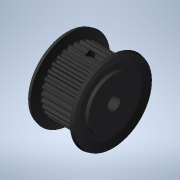
# Autodesk Inventor part: HTPA32S2M100-A-P4_a
Saved by Autodesk Inventor 2021 (Build 250183000, 183)
## iProperties
Created: 2025-04-04
Part Number: HTPA32S2M100-A-P4_a
Material: Generic
Catalog Web Link: www.cadenas.de
Description: HTPA_ _S2M040, HTPA_ _S2M060, HTPA_ _S2M100, HTPB_ _S2M040, HTPB_ _S2M060, HTPB_ _S2M100, HTPK_ _S2M040, HTPK_ _S2M060, HTPK_ _S2M100, HTPN_ _S2M040, HTPN_ _S2M060, HTPN_ _S2M100, HTPT_ _S2M040, HTPT_ _S2M060, HTPM_ _S2M040, HTPM_ _S2M060, HTPP_ _S2M040, HTPP_ _S2M060, HTPS_ _S2M040, HTPS_ _S2M060, HTPS_ _S2M100_a-High Torque Timing Pulleys S2M Type
Vendor: MISUMI
Document SubType Name: Modeling
Designer: psAdmin
Manufacturer: MISUMI
Mass: 4.25657 g
Surface Area: 28.5328 cm^2
Volume: 4.25657 cm^3
Density: 1 g/cm^3
Appearance: PSOLRGB-175-175-175
Category: PARTsolutions
Company: MISUMI
Title: HTPA32S2M100-A-P4
Author: Cadenas PARTsolutions
Comments: High Torque Timing Pulleys S2M Type
PSOL_IDENT_0: {$CADENAS_DATA/23d-libs/misumi/metric/51_timing_pulleys/htpm_s2m/htpa_s2m.prj},735 {VTYP=3D},{NB=HTP
PSOL_IDENT_1: A32S2M100-A-P4_a},{LINA=HTPA32S2M100-A-P4},{NN=HTPA_ _S2M040, HTPA_ _S2M060, HTPA_ _S2M100, HTPB_ _S
PSOL_IDENT_2: 2M040, HTPB_ _S2M060, HTPB_ _S2M100, HTPK_ _S2M040, HTPK_ _S2M060, HTPK_ _S2M100, HTPN_ _S2M040, HTP
PSOL_IDENT_3: N_ _S2M060, HTPN_ _S2M100, HTPT_ _S2M040, HTPT_ _S2M060, HTPM_ _S2M040, HTPM_ _S2M060, HTPP_ _S2M040
PSOL_IDENT_4: , HTPP_ _S2M060, HTPS_ _S2M040, HTPS_ _S2M060, HTPS_ _S2M100_a},{DATE=29.05.2023 09:16:33},{GEOMDATE=
PSOL_IDENT_5: 11.01.2023 01:57:31},{VERSION=},{LINEID=170},{WBVAR=MATP,ST,TNW,PS,SBS,DD,Z,J,Q,R,S,T,ALT1,ALT2,M,QS
PSOL_IDENT_6: C,QFC,QTC,ALT3,K,KSC,KFC,KTC,ALT4,ZM,ZSC,ZFC,ZTC,ALT5,ALT6,ALT7,FC,ALT8,SRG,ALT9,BTC,TL,ALT10,TPC,AL
PSOL_IDENT_7: T11,BC,ALT12,SLH,ALT13,BN},{WBNUMERIC=DD,Z,J,Q,R,S,T,QSC,QFC,QTC,K,KSC,KFC,KTC,ZSC,ZFC,ZTC,FC,SRG,BT
PSOL_IDENT_8: C,TL,BC,SLH,BN}  {NB=HTPA32S2M100-A-P4_a},{LINA=HTPA32S2M100-A-P4},{KT=DUMMY},{PN=HTPA32S2M100-A-P4}
PSOL_IDENT_9: ,{TYPE=HTPA},{MATP=A2017},{MATPALG= 'A2017','Aluminum Alloy 2000 series','S45CE','1045 Carbon Steel
PSOL_IDENT_10: Equivalent','SUS304','304 Stainless Steel' },{ST=CA},{STALG= 'CA' , 'Clear Anodize', 'BA','Black Ano
PSOL_IDENT_11: dize','HAT','Hard Clear Anodize' , 'ENP' , 'Electroless Nickel Plating' },{NT=32},{TNW=S2M100},{TNWA
PSOL_IDENT_12: LG= 'S2M040', 'S2M060','S2M100' },{BW=10},{PS=A},{PSALG='A','B'},{SBS=P},{SBSALG= 'H','Round Hole','
PSOL_IDENT_13: P','Round Hole + Tap','N','New JIS Keywayed Bore + Tap (Standard)','V','Stepped Hole','Y','Both Ends
PSOL_IDENT_14: Stepped Hole','WB','Double Stepped Hole' },{SHSA= 'H','Round Hole','P','Round Hole + Tap','N','New
PSOL_IDENT_15: JIS Keywayed Bore + Tap (Standard)','V','Stepped Hole','Y','Both Ends Stepped Hole','WB','Double Ste
PSOL_IDENT_16: pped Hole' },{SHSB='H','Round Hole','P','Round Hole + Tap','V','Stepped Hole','F','Stepped Hole (Cou
PSOL_IDENT_17: nterbore holes on the boss side)' },{SHSK='H','Round Hole','P','Round Hole + Tap'},{SBSPN=-P4},{DD=4
PSOL_IDENT_18: .00},{DDALG=[4:4/1],4.5,[5:6/1],6.35,[7:10/1]},{DDHA=[4:4/1],4.5,[5:6/1],6.35,[7:12/1]},{DDHBK=0},{D
PSOL_IDENT_19: DPA=[4:4/1],4.5,[5:6/1],6.35,[7:10/1]},{DDPBK=0},{DDNA=[8:8/1]},{DDNBK=0},{DDNK=0},{DDCA=0},{DDCBK=0
PSOL_IDENT_20: },{DDVA=[4:4/1],4.5,[5:6/1],6.35,[7:10/1]},{DDVF=0},{DDY=[4:10/1]},{DDWB=[4:8/1]},{Z=0},{ZALG=[0]},{
PSOL_IDENT_21: ZQRMIN=6},{ZAMAX=12},{ZBMAX=0},{DDZ=4},{J=0.0},{JALG=[0]},{JMAX=13},{JMIN=2},{JPN=},{QRMAX=12},{QRMI
PSOL_IDENT_22: N=6},{WBRMAX=-2.00},{WBQMIN=8},{Q=0},{QALG=[0]},{QPN=},{R=0},{RALG=[0]},{S=0.0},{SALG=[0]},{SPN=},{S
PSOL_IDENT_23: MAX=9},{T=0.0},{TALG=[0]},{TPN=},{TMAX=12},{A=11},{W=15},{L=0},{PD=20.37},{OD=19.86},{D=0},{DALG=12}
PSOL_IDENT_24: ,{DE=16},{F=25},{E=16},{BBK=0.000},{TTK=0.0},{TT=1},{WL=15.000},{ALT1=},{ALT1ALG= '','w/o KC90 (Set
PSOL_IDENT_25: Screw Angle)','KC90','with KC90 (Set Screw Angle)' },{ANG=123.750},{ALT1PN=},{ALT2=},{ALT2ALG= '','N
PSOL_IDENT_26: ot applicable' },{M=N/A},{MALG= 'N/A' },{MFTALG= 'N/A' },{MSALG= 'N/A' },{M3D=0.000},{KDML=0},{ML=0}
PSOL_IDENT_27: ,{MUL=0},{PITCH=0},{QSC=0.0},{QSCALG=0},{QFC=0.0},{QFCALG=0},{QTC=0.0},{QTCALG=0},{QPCDMIN=0},{QPCDM
PSOL_IDENT_28: INALG=0},{QPCDMAX=12},{ALT2PN=},{ALT3=},{ALT3ALG= '','Not applicable' },{K=0.0},{KALG=0},{KMIN=4},{K
PSOL_IDENT_29: FTMAX=0.0},{KSMAX=0.0},{KSC=0.0},{KSCALG=0},{KFC=0.0},{KFCALG=0},{KTC=0.0},{KTCALG=0},{KPCDMIN=8},{K
PSOL_IDENT_30: PCDMINALG=8},{KPCDMAX=12},{KSCMIN=8.0},{KSCMINALG=8},{ALT3PN=},{ALT4=},{ALT4ALG= '','Not applicable'
PSOL_IDENT_31: },{ALT4MIN=14.5},{ALT4MAX=5.5},{ZM=N/A},{ZMALG= 'N/A' },{ZMSALG= 'N/A' },{ZMFTALG= 'N/A' },{ZMDD1=0
PSOL_IDENT_32: .0},{ZMDD2=0.0},{ZMHH=0.0},{ZSC=0.0},{ZSCALG=[0]},{ZFC=0.0},{ZFCALG=[0]},{ZTC=0.0},{ZTCALG=[0]},{ZPC
PSOL_IDENT_33: DMIN=0},{ZPCDMINALG=0},{ZPCDMAX=12},{ALT4PN=},{ALT5=},{ALT5ALG= '','Flange Attached','NFC','with NFC
PSOL_IDENT_34: (Flange not Attached)' },{ALT5PN=},{ALT6=},{ALT6ALG= '','w/o Flange Attached on One Side Only','RFC'
PSOL_IDENT_35: ,'with RFC (Flange Attached on The Boss Side Only)','LFC','with LFC (Flange Attached on The Opposite
PSOL_IDENT_36: Side Only)' },{ALT6PN=},{ALT7=},{ALT7ALG= '','w/o FC (Flange Cut)','FC','with FC (Flange Cut)' },{F
PSOL_IDENT_37: C=0.0},{FCALG=0},{FCMIN=21.0},{FCMAX=23.0},{ALT7PN=},{ALT8=},{ALT8ALG= '','Not applicable' },{ALT8AL
PSOL_IDENT_38: GALG=12},{ALT8DD2=0},{ALT8MM=0},{ALT8NN=0},{QC=0},{KC=0},{ZC=0},{SRG=0.0},{SRGALG=[0]},{SRGMAX=0},{D
PSOL_IDENT_39: D2=0.0},{MM=0.00},{NN=0.00},{ALT8PN=},{ALT9ALG= '','w/o BTC (Taper for Bearing Holder)','BTC','with
PSOL_IDENT_40: BTC (Taper for Bearing Holder)' },{ALT9=},{BTC9=6},{TL9=1},{BTC=0},{BTCALG=[0]},{TL=0.0},{TLALG=[0]}
PSOL_IDENT_41: ,{TLMIN=1.0},{TLMAX=-15.5},{BTCL=0},{BTCD=0},{BTCDALG=12.000},{ALT9PN=},{WLBCTL=15},{ALT10=},{ALT10A
PSOL_IDENT_42: LG= '','w/o TPC (Tapped Hole Dimension)','TPC','with TPC (Tapped Hole Dimension)' },{TPC=N/A},{TPCAL
PSOL_IDENT_43: G= 'N/A' },{TPCM=3},{ALT10PN=},{ALT11=},{ALT11ALG= '','Not applicable' },{BC=0.0},{BCALG=0},{BCMIN=6
PSOL_IDENT_44: },{BCMAX=-15.5},{BCPLANE=7.5},{M1WBC=7.5},{ALT11PN=},{ALT12=},{ALT12ALG= '','w/o SLH (Set Screw Leng
PSOL_IDENT_45: th)','SLH','with SLH (Set Screw Length)' },{SLH=0},{SLHALG=[0]},{ALT12PN=},{ALT13=},{ALT13ALG= '', '
PSOL_IDENT_46: Not applicable' },{BN=0.0},{BNALG=0},{BNMIN=-14.5},{BNMAX=-5},{ALT13PN=},{AC=M3x3},{M1=3},{M1L=3},{T
PSOL_IDENT_47: AP=0.000},{KYY=2},{KTT=7.93},{PLANE=15},{CD=0},{SRGCUT=1}
NB: HTPA32S2M100-A-P4_a
NN: HTPA_ _S2M040, HTPA_ _S2M060, HTPA_ _S2M100, HTPB_ _S2M040, HTPB_ _S2M060, HTPB_ _S2M100, HTPK_ _S2M040, HTPK_ _S2M060, HTPK_ _S2M100, HTPN_ _S2M040, HTPN_ _S2M060, HTPN_ _S2M100, HTPT_ _S2M040, HTPT_ _S2M060, HTPM_ _S2M040, HTPM_ _S2M060, HTPP_ _S2M040, HTPP_ _S2M060, HTPS_ _S2M040, HTPS_ _S2M060, HTPS_ _S2M100_a
NT: 32
NBSYN: $PN._a
LINA: HTPA32S2M100-A-P4
CATALOG: Misumi
PN: HTPA32S2M100-A-P4
MATP: Aluminum Alloy 2000 series
ST: Clear Anodize
TNW: S2M100
BW: 10
PS: A
SBS: Round Hole + Tap
DD: 4
Z: 0
J: 0
Q: 0
R: 0
S: 0
T: 0
A: 11
W: 15
L: 0
PD: 20.37
OD: 19.86
D: 0
F: 25
ALT1: w/o KC90 (Set Screw Angle)
ALT2: Not applicable
M: N/A
QSC: 0
QFC: 0
QTC: 0
ALT3: Not applicable
K: 0
KSC: 0
KFC: 0
KTC: 0
ALT4: Not applicable
ZM: N/A
ZSC: 0
ZFC: 0
ZTC: 0
ALT5: Flange Attached
ALT6: w/o Flange Attached on One Side Only
ALT7: w/o FC (Flange Cut)
FC: 0
ALT8: Not applicable
SRG: 0
ALT9: w/o BTC (Taper for Bearing Holder)
BTC: 0
TL: 0
ALT10: w/o TPC (Tapped Hole Dimension)
TPC: N/A
ALT11: Not applicable
BC: 0
ALT12: w/o SLH (Set Screw Length)
SLH: 0
ALT13: Not applicable
BN: 0
AC: M3x3
SUPPLIER: MISUMI
ARTICLENO: HTPA32S2M100-A-P4_a
BOMINFO: HTPA32S2M100-A-P4
CREATOR: CADENAS GmbH
Autodesk Inventor part; units mm, degrees
ref_plane "YZ Plane" through (0, 0, 0) normal (1, 0, 0) x (0, 1, 0)
ref_plane "XZ Plane" through (0, 0, 0) normal (0, 1, 0) x (-1, 0, 0)
ref_plane "XY Plane" through (0, 0, 0) normal (0, 0, 1) x (1, 0, 0)
sketch "_____1" plane through (0, 0, 0) normal (0, 0, 1) x (1, 0, 0)
  line L0 (15, 0) -> (0, 0)
  line L1 (0, 0) -> (0, 8)
  line L2 (0, 8) -> (1, 8)
  line L3 (1, 8) -> (1, 9.7983)
  line L4 (1, 9.7983) -> (0.3454, 12.2412)
  line L5 (0.3454, 12.2412) -> (1.3114, 12.5)
  line L6 (1.3114, 12.5) -> (2, 9.93)
  line L7 (2, 9.93) -> (13, 9.93)
  line L8 (13, 9.93) -> (13.6886, 12.5)
  line L9 (13.6886, 12.5) -> (14.6546, 12.2412)
  line L10 (14.6546, 12.2412) -> (14, 9.7983)
  line L11 (14, 9.7983) -> (14, 8)
  line L12 (14, 8) -> (15, 8)
  line L13 (15, 8) -> (15, 0)
  line L14 (15, 0) -> (0, 0)
  constraints: 30 end point
revolve "Revolution1" add sketch "_____1" angle 360 about axis through (15, 0, 0) along (1, 0, 0)
sketch "Sketch2" plane through (15, 0, 0) normal (1, 0, 0) x (0, 0, -1)
  point P0 (0, 0)
hole "Hole1" at (15, 0, 0) direction (-1, 0, 0) diameter 4 depth 15
sketch "_____6" plane through (2, 0, 0) normal (1, 0, 0) x (0, 0, -1)
  circle A0 centre (0, 0) radius 19.86
  arc A1 (-9.7648, -0.6134) -> (-9.8969, -0.81) centre (-9.7075, -0.7945) ccw
  arc A2 (-9.8969, -0.81) -> (-9.8822, -0.9733) centre (0, 0) ccw
  arc A3 (-9.8822, -0.9733) -> (-9.8648, -1.1363) centre (0, 0) ccw
  arc A4 (-9.8648, -1.1363) -> (-9.6968, -1.3034) centre (-9.676, -1.1146) ccw
  arc A5 (-9.0678, -1.5453) -> (-9.6968, -1.3034) centre (-9.8421, -2.6205) ccw
  arc A6 (-9.0278, -1.6089) -> (-9.0678, -1.5453) centre (-9.1262, -1.6264) ccw
  arc A7 (-9.0278, -1.6089) -> (-8.9563, -1.9684) centre (0, 0) ccw
  arc A8 (-8.9689, -2.0424) -> (-8.9563, -1.9684) centre (-9.0539, -1.9898) ccw
  arc A9 (-9.4575, -2.5066) -> (-8.9689, -2.0424) centre (-10.0957, -1.3454) ccw
  arc A10 (-9.4575, -2.5066) -> (-9.5487, -2.7253) centre (-9.366, -2.6731) ccw
  arc A11 (-9.5487, -2.7253) -> (-9.5024, -2.8825) centre (0, 0) ccw
  arc A12 (-9.5024, -2.8825) -> (-9.4535, -3.039) centre (0, 0) ccw
  arc A13 (-9.4535, -3.039) -> (-9.2562, -3.1702) centre (-9.2726, -2.9809) ccw
  arc A14 (-8.5921, -3.2846) -> (-9.2562, -3.1702) centre (-9.1418, -4.4902) ccw
  arc A15 (-8.5404, -3.3392) -> (-8.5921, -3.2846) centre (-8.6335, -3.3756) ccw
  arc A16 (-8.5404, -3.3392) -> (-8.4002, -3.6778) centre (0, 0) ccw
  arc A17 (-8.3981, -3.7529) -> (-8.4002, -3.6778) centre (-8.4918, -3.7179) ccw
  arc A18 (-8.7868, -4.3035) -> (-8.3981, -3.7529) centre (-9.6393, -3.2892) ccw
  arc A19 (-8.7868, -4.3035) -> (-8.8336, -4.5357) centre (-8.6645, -4.449) ccw
  arc A20 (-8.8336, -4.5357) -> (-8.7575, -4.681) centre (0, 0) ccw
  arc A21 (-8.7575, -4.681) -> (-8.679, -4.8249) centre (0, 0) ccw
  arc A22 (-8.679, -4.8249) -> (-8.4599, -4.915) centre (-8.5129, -4.7326) ccw
  arc A23 (-7.7862, -4.8977) -> (-8.4599, -4.915) centre (-8.0901, -6.1874) ccw
  arc A24 (-7.7249, -4.9412) -> (-7.7862, -4.8977) centre (-7.8091, -4.9951) ccw
  arc A25 (-7.7249, -4.9412) -> (-7.5212, -5.2459) centre (0, 0) ccw
  arc A26 (-7.5046, -5.3192) -> (-7.5212, -5.2459) centre (-7.6033, -5.3031) ccw
  arc A27 (-7.7784, -5.935) -> (-7.5046, -5.3192) centre (-8.8124, -5.1065) ccw
  arc A28 (-7.7784, -5.935) -> (-7.779, -6.1719) centre (-7.6301, -6.0538) ccw
  arc A29 (-7.779, -6.1719) -> (-7.676, -6.2995) centre (0, 0) ccw
  arc A30 (-7.676, -6.2995) -> (-7.5709, -6.4254) centre (0, 0) ccw
  arc A31 (-7.5709, -6.4254) -> (-7.3385, -6.4711) centre (-7.4261, -6.3025) ccw
  arc A32 (-6.6811, -6.3226) -> (-7.3385, -6.4711) centre (-6.7276, -7.6468) ccw
  arc A33 (-6.6125, -6.3533) -> (-6.6811, -6.3226) centre (-6.6846, -6.4226) ccw
  arc A34 (-6.6125, -6.3533) -> (-6.3533, -6.6125) centre (0, 0) ccw
  arc A35 (-6.3226, -6.6811) -> (-6.3533, -6.6125) centre (-6.4226, -6.6846) ccw
  arc A36 (-6.4711, -7.3385) -> (-6.3226, -6.6811) centre (-7.6468, -6.7276) ccw
  arc A37 (-6.4711, -7.3385) -> (-6.4254, -7.5709) centre (-6.3025, -7.4261) ccw
  arc A38 (-6.4254, -7.5709) -> (-6.2995, -7.676) centre (0, 0) ccw
  arc A39 (-6.2995, -7.676) -> (-6.1719, -7.779) centre (0, 0) ccw
  arc A40 (-6.1719, -7.779) -> (-5.935, -7.7784) centre (-6.0538, -7.6301) ccw
  arc A41 (-5.3192, -7.5046) -> (-5.935, -7.7784) centre (-5.1065, -8.8124) ccw
  arc A42 (-5.2459, -7.5212) -> (-5.3192, -7.5046) centre (-5.3031, -7.6033) ccw
  arc A43 (-5.2459, -7.5212) -> (-4.9412, -7.7249) centre (0, 0) ccw
  arc A44 (-4.8977, -7.7862) -> (-4.9412, -7.7249) centre (-4.9951, -7.8091) ccw
  arc A45 (-4.915, -8.4599) -> (-4.8977, -7.7862) centre (-6.1874, -8.0901) ccw
  arc A46 (-4.915, -8.4599) -> (-4.8249, -8.679) centre (-4.7326, -8.5129) ccw
  arc A47 (-4.8249, -8.679) -> (-4.681, -8.7575) centre (0, 0) ccw
  arc A48 (-4.681, -8.7575) -> (-4.5357, -8.8336) centre (0, 0) ccw
  arc A49 (-4.5357, -8.8336) -> (-4.3035, -8.7868) centre (-4.449, -8.6645) ccw
  arc A50 (-3.7529, -8.3981) -> (-4.3035, -8.7868) centre (-3.2892, -9.6393) ccw
  arc A51 (-3.6778, -8.4002) -> (-3.7529, -8.3981) centre (-3.7179, -8.4918) ccw
  arc A52 (-3.6778, -8.4002) -> (-3.3392, -8.5404) centre (0, 0) ccw
  arc A53 (-3.2846, -8.5921) -> (-3.3392, -8.5404) centre (-3.3756, -8.6335) ccw
  arc A54 (-3.1702, -9.2562) -> (-3.2846, -8.5921) centre (-4.4902, -9.1418) ccw
  arc A55 (-3.1702, -9.2562) -> (-3.039, -9.4535) centre (-2.9809, -9.2726) ccw
  arc A56 (-3.039, -9.4535) -> (-2.8825, -9.5024) centre (0, 0) ccw
  arc A57 (-2.8825, -9.5024) -> (-2.7253, -9.5487) centre (0, 0) ccw
  arc A58 (-2.7253, -9.5487) -> (-2.5066, -9.4575) centre (-2.6731, -9.366) ccw
  arc A59 (-2.0424, -8.9689) -> (-2.5066, -9.4575) centre (-1.3454, -10.0957) ccw
  arc A60 (-1.9684, -8.9563) -> (-2.0424, -8.9689) centre (-1.9898, -9.0539) ccw
  arc A61 (-1.9684, -8.9563) -> (-1.6089, -9.0278) centre (0, 0) ccw
  arc A62 (-1.5453, -9.0678) -> (-1.6089, -9.0278) centre (-1.6264, -9.1262) ccw
  arc A63 (-1.3034, -9.6968) -> (-1.5453, -9.0678) centre (-2.6205, -9.8421) ccw
  arc A64 (-1.3034, -9.6968) -> (-1.1363, -9.8648) centre (-1.1146, -9.676) ccw
  arc A65 (-1.1363, -9.8648) -> (-0.9733, -9.8822) centre (0, 0) ccw
  arc A66 (-0.9733, -9.8822) -> (-0.81, -9.8969) centre (0, 0) ccw
  arc A67 (-0.81, -9.8969) -> (-0.6134, -9.7648) centre (-0.7945, -9.7075) ccw
  arc A68 (-0.2534, -9.195) -> (-0.6134, -9.7648) centre (0.65, -10.1642) ccw
  arc A69 (-0.1833, -9.1682) -> (-0.2534, -9.195) centre (-0.1853, -9.2681) ccw
  arc A70 (-0.1833, -9.1682) -> (0.1833, -9.1682) centre (0, 0) ccw
  arc A71 (0.2534, -9.195) -> (0.1833, -9.1682) centre (0.1853, -9.2681) ccw
  arc A72 (0.6134, -9.7648) -> (0.2534, -9.195) centre (-0.65, -10.1642) ccw
  arc A73 (0.6134, -9.7648) -> (0.81, -9.8969) centre (0.7945, -9.7075) ccw
  arc A74 (0.81, -9.8969) -> (0.9733, -9.8822) centre (0, 0) ccw
  arc A75 (0.9733, -9.8822) -> (1.1363, -9.8648) centre (0, 0) ccw
  arc A76 (1.1363, -9.8648) -> (1.3034, -9.6968) centre (1.1146, -9.676) ccw
  arc A77 (1.5453, -9.0678) -> (1.3034, -9.6968) centre (2.6205, -9.8421) ccw
  arc A78 (1.6089, -9.0278) -> (1.5453, -9.0678) centre (1.6264, -9.1262) ccw
  arc A79 (1.6089, -9.0278) -> (1.9684, -8.9563) centre (0, 0) ccw
  arc A80 (2.0424, -8.9689) -> (1.9684, -8.9563) centre (1.9898, -9.0539) ccw
  arc A81 (2.5066, -9.4575) -> (2.0424, -8.9689) centre (1.3454, -10.0957) ccw
  arc A82 (2.5066, -9.4575) -> (2.7253, -9.5487) centre (2.6731, -9.366) ccw
  arc A83 (2.7253, -9.5487) -> (2.8825, -9.5024) centre (0, 0) ccw
  arc A84 (2.8825, -9.5024) -> (3.039, -9.4535) centre (0, 0) ccw
  arc A85 (3.039, -9.4535) -> (3.1702, -9.2562) centre (2.9809, -9.2726) ccw
  arc A86 (3.2846, -8.5921) -> (3.1702, -9.2562) centre (4.4902, -9.1418) ccw
  arc A87 (3.3392, -8.5404) -> (3.2846, -8.5921) centre (3.3756, -8.6335) ccw
  arc A88 (3.3392, -8.5404) -> (3.6778, -8.4002) centre (0, 0) ccw
  arc A89 (3.7529, -8.3981) -> (3.6778, -8.4002) centre (3.7179, -8.4918) ccw
  arc A90 (4.3035, -8.7868) -> (3.7529, -8.3981) centre (3.2892, -9.6393) ccw
  arc A91 (4.3035, -8.7868) -> (4.5357, -8.8336) centre (4.449, -8.6645) ccw
  arc A92 (4.5357, -8.8336) -> (4.681, -8.7575) centre (0, 0) ccw
  arc A93 (4.681, -8.7575) -> (4.8249, -8.679) centre (0, 0) ccw
  arc A94 (4.8249, -8.679) -> (4.915, -8.4599) centre (4.7326, -8.5129) ccw
  arc A95 (4.8977, -7.7862) -> (4.915, -8.4599) centre (6.1874, -8.0901) ccw
  arc A96 (4.9412, -7.7249) -> (4.8977, -7.7862) centre (4.9951, -7.8091) ccw
  arc A97 (4.9412, -7.7249) -> (5.2459, -7.5212) centre (0, 0) ccw
  arc A98 (5.3192, -7.5046) -> (5.2459, -7.5212) centre (5.3031, -7.6033) ccw
  arc A99 (5.935, -7.7784) -> (5.3192, -7.5046) centre (5.1065, -8.8124) ccw
  arc A100 (5.935, -7.7784) -> (6.1719, -7.779) centre (6.0538, -7.6301) ccw
  arc A101 (6.1719, -7.779) -> (6.2995, -7.676) centre (0, 0) ccw
  arc A102 (6.2995, -7.676) -> (6.4254, -7.5709) centre (0, 0) ccw
  arc A103 (6.4254, -7.5709) -> (6.4711, -7.3385) centre (6.3025, -7.4261) ccw
  arc A104 (6.3226, -6.6811) -> (6.4711, -7.3385) centre (7.6468, -6.7276) ccw
  arc A105 (6.3533, -6.6125) -> (6.3226, -6.6811) centre (6.4226, -6.6846) ccw
  arc A106 (6.3533, -6.6125) -> (6.6125, -6.3533) centre (0, 0) ccw
  arc A107 (6.6811, -6.3226) -> (6.6125, -6.3533) centre (6.6846, -6.4226) ccw
  arc A108 (7.3385, -6.4711) -> (6.6811, -6.3226) centre (6.7276, -7.6468) ccw
  arc A109 (7.3385, -6.4711) -> (7.5709, -6.4254) centre (7.4261, -6.3025) ccw
  arc A110 (7.5709, -6.4254) -> (7.676, -6.2995) centre (0, 0) ccw
  arc A111 (7.676, -6.2995) -> (7.779, -6.1719) centre (0, 0) ccw
  arc A112 (7.779, -6.1719) -> (7.7784, -5.935) centre (7.6301, -6.0538) ccw
  arc A113 (7.5046, -5.3192) -> (7.7784, -5.935) centre (8.8124, -5.1065) ccw
  arc A114 (7.5212, -5.2459) -> (7.5046, -5.3192) centre (7.6033, -5.3031) ccw
  arc A115 (7.5212, -5.2459) -> (7.7249, -4.9412) centre (0, 0) ccw
  arc A116 (7.7862, -4.8977) -> (7.7249, -4.9412) centre (7.8091, -4.9951) ccw
  arc A117 (8.4599, -4.915) -> (7.7862, -4.8977) centre (8.0901, -6.1874) ccw
  arc A118 (8.4599, -4.915) -> (8.679, -4.8249) centre (8.5129, -4.7326) ccw
  arc A119 (8.679, -4.8249) -> (8.7575, -4.681) centre (0, 0) ccw
  arc A120 (8.7575, -4.681) -> (8.8336, -4.5357) centre (0, 0) ccw
  arc A121 (8.8336, -4.5357) -> (8.7868, -4.3035) centre (8.6645, -4.449) ccw
  arc A122 (8.3981, -3.7529) -> (8.7868, -4.3035) centre (9.6393, -3.2892) ccw
  arc A123 (8.4002, -3.6778) -> (8.3981, -3.7529) centre (8.4918, -3.7179) ccw
  arc A124 (8.4002, -3.6778) -> (8.5404, -3.3392) centre (0, 0) ccw
  arc A125 (8.5921, -3.2846) -> (8.5404, -3.3392) centre (8.6335, -3.3756) ccw
  arc A126 (9.2562, -3.1702) -> (8.5921, -3.2846) centre (9.1418, -4.4902) ccw
  arc A127 (9.2562, -3.1702) -> (9.4535, -3.039) centre (9.2726, -2.9809) ccw
  arc A128 (9.4535, -3.039) -> (9.5024, -2.8825) centre (0, 0) ccw
  arc A129 (9.5024, -2.8825) -> (9.5487, -2.7253) centre (0, 0) ccw
  arc A130 (9.5487, -2.7253) -> (9.4575, -2.5066) centre (9.366, -2.6731) ccw
  arc A131 (8.9689, -2.0424) -> (9.4575, -2.5066) centre (10.0957, -1.3454) ccw
  arc A132 (8.9563, -1.9684) -> (8.9689, -2.0424) centre (9.0539, -1.9898) ccw
  arc A133 (8.9563, -1.9684) -> (9.0278, -1.6089) centre (0, 0) ccw
  arc A134 (9.0678, -1.5453) -> (9.0278, -1.6089) centre (9.1262, -1.6264) ccw
  arc A135 (9.6968, -1.3034) -> (9.0678, -1.5453) centre (9.8421, -2.6205) ccw
  arc A136 (9.6968, -1.3034) -> (9.8648, -1.1363) centre (9.676, -1.1146) ccw
  arc A137 (9.8648, -1.1363) -> (9.8822, -0.9733) centre (0, 0) ccw
  arc A138 (9.8822, -0.9733) -> (9.8969, -0.81) centre (0, 0) ccw
  arc A139 (9.8969, -0.81) -> (9.7648, -0.6134) centre (9.7075, -0.7945) ccw
  arc A140 (9.195, -0.2534) -> (9.7648, -0.6134) centre (10.1642, 0.65) ccw
  arc A141 (9.1682, -0.1833) -> (9.195, -0.2534) centre (9.2681, -0.1853) ccw
  arc A142 (9.1682, -0.1833) -> (9.1682, 0.1833) centre (0, 0) ccw
  arc A143 (9.195, 0.2534) -> (9.1682, 0.1833) centre (9.2681, 0.1853) ccw
  arc A144 (9.7648, 0.6134) -> (9.195, 0.2534) centre (10.1642, -0.65) ccw
  arc A145 (9.7648, 0.6134) -> (9.8969, 0.81) centre (9.7075, 0.7945) ccw
  arc A146 (9.8969, 0.81) -> (9.8822, 0.9733) centre (0, 0) ccw
  arc A147 (9.8822, 0.9733) -> (9.8648, 1.1363) centre (0, 0) ccw
  arc A148 (9.8648, 1.1363) -> (9.6968, 1.3034) centre (9.676, 1.1146) ccw
  arc A149 (9.0678, 1.5453) -> (9.6968, 1.3034) centre (9.8421, 2.6205) ccw
  arc A150 (9.0278, 1.6089) -> (9.0678, 1.5453) centre (9.1262, 1.6264) ccw
  arc A151 (9.0278, 1.6089) -> (8.9563, 1.9684) centre (0, 0) ccw
  arc A152 (8.9689, 2.0424) -> (8.9563, 1.9684) centre (9.0539, 1.9898) ccw
  arc A153 (9.4575, 2.5066) -> (8.9689, 2.0424) centre (10.0957, 1.3454) ccw
  arc A154 (9.4575, 2.5066) -> (9.5487, 2.7253) centre (9.366, 2.6731) ccw
  arc A155 (9.5487, 2.7253) -> (9.5024, 2.8825) centre (0, 0) ccw
  arc A156 (9.5024, 2.8825) -> (9.4535, 3.039) centre (0, 0) ccw
  arc A157 (9.4535, 3.039) -> (9.2562, 3.1702) centre (9.2726, 2.9809) ccw
  arc A158 (8.5921, 3.2846) -> (9.2562, 3.1702) centre (9.1418, 4.4902) ccw
  arc A159 (8.5404, 3.3392) -> (8.5921, 3.2846) centre (8.6335, 3.3756) ccw
  arc A160 (8.5404, 3.3392) -> (8.4002, 3.6778) centre (0, 0) ccw
  arc A161 (8.3981, 3.7529) -> (8.4002, 3.6778) centre (8.4918, 3.7179) ccw
  arc A162 (8.7868, 4.3035) -> (8.3981, 3.7529) centre (9.6393, 3.2892) ccw
  arc A163 (8.7868, 4.3035) -> (8.8336, 4.5357) centre (8.6645, 4.449) ccw
  arc A164 (8.8336, 4.5357) -> (8.7575, 4.681) centre (0, 0) ccw
  arc A165 (8.7575, 4.681) -> (8.679, 4.8249) centre (0, 0) ccw
  arc A166 (8.679, 4.8249) -> (8.4599, 4.915) centre (8.5129, 4.7326) ccw
  arc A167 (7.7862, 4.8977) -> (8.4599, 4.915) centre (8.0901, 6.1874) ccw
  arc A168 (7.7249, 4.9412) -> (7.7862, 4.8977) centre (7.8091, 4.9951) ccw
  arc A169 (7.7249, 4.9412) -> (7.5212, 5.2459) centre (0, 0) ccw
  arc A170 (7.5046, 5.3192) -> (7.5212, 5.2459) centre (7.6033, 5.3031) ccw
  arc A171 (7.7784, 5.935) -> (7.5046, 5.3192) centre (8.8124, 5.1065) ccw
  arc A172 (7.7784, 5.935) -> (7.779, 6.1719) centre (7.6301, 6.0538) ccw
  arc A173 (7.779, 6.1719) -> (7.676, 6.2995) centre (0, 0) ccw
  arc A174 (7.676, 6.2995) -> (7.5709, 6.4254) centre (0, 0) ccw
  arc A175 (7.5709, 6.4254) -> (7.3385, 6.4711) centre (7.4261, 6.3025) ccw
  arc A176 (6.6811, 6.3226) -> (7.3385, 6.4711) centre (6.7276, 7.6468) ccw
  arc A177 (6.6125, 6.3533) -> (6.6811, 6.3226) centre (6.6846, 6.4226) ccw
  arc A178 (6.6125, 6.3533) -> (6.3533, 6.6125) centre (0, 0) ccw
  arc A179 (6.3226, 6.6811) -> (6.3533, 6.6125) centre (6.4226, 6.6846) ccw
  arc A180 (6.4711, 7.3385) -> (6.3226, 6.6811) centre (7.6468, 6.7276) ccw
  arc A181 (6.4711, 7.3385) -> (6.4254, 7.5709) centre (6.3025, 7.4261) ccw
  arc A182 (6.4254, 7.5709) -> (6.2995, 7.676) centre (0, 0) ccw
  arc A183 (6.2995, 7.676) -> (6.1719, 7.779) centre (0, 0) ccw
  arc A184 (6.1719, 7.779) -> (5.935, 7.7784) centre (6.0538, 7.6301) ccw
  arc A185 (5.3192, 7.5046) -> (5.935, 7.7784) centre (5.1065, 8.8124) ccw
  arc A186 (5.2459, 7.5212) -> (5.3192, 7.5046) centre (5.3031, 7.6033) ccw
  arc A187 (5.2459, 7.5212) -> (4.9412, 7.7249) centre (0, 0) ccw
  arc A188 (4.8977, 7.7862) -> (4.9412, 7.7249) centre (4.9951, 7.8091) ccw
  arc A189 (4.915, 8.4599) -> (4.8977, 7.7862) centre (6.1874, 8.0901) ccw
  arc A190 (4.915, 8.4599) -> (4.8249, 8.679) centre (4.7326, 8.5129) ccw
  arc A191 (4.8249, 8.679) -> (4.681, 8.7575) centre (0, 0) ccw
  arc A192 (4.681, 8.7575) -> (4.5357, 8.8336) centre (0, 0) ccw
  arc A193 (4.5357, 8.8336) -> (4.3035, 8.7868) centre (4.449, 8.6645) ccw
  arc A194 (3.7529, 8.3981) -> (4.3035, 8.7868) centre (3.2892, 9.6393) ccw
  arc A195 (3.6778, 8.4002) -> (3.7529, 8.3981) centre (3.7179, 8.4918) ccw
  arc A196 (3.6778, 8.4002) -> (3.3392, 8.5404) centre (0, 0) ccw
  arc A197 (3.2846, 8.5921) -> (3.3392, 8.5404) centre (3.3756, 8.6335) ccw
  arc A198 (3.1702, 9.2562) -> (3.2846, 8.5921) centre (4.4902, 9.1418) ccw
  arc A199 (3.1702, 9.2562) -> (3.039, 9.4535) centre (2.9809, 9.2726) ccw
  arc A200 (3.039, 9.4535) -> (2.8825, 9.5024) centre (0, 0) ccw
  arc A201 (2.8825, 9.5024) -> (2.7253, 9.5487) centre (0, 0) ccw
  arc A202 (2.7253, 9.5487) -> (2.5066, 9.4575) centre (2.6731, 9.366) ccw
  arc A203 (2.0424, 8.9689) -> (2.5066, 9.4575) centre (1.3454, 10.0957) ccw
  arc A204 (1.9684, 8.9563) -> (2.0424, 8.9689) centre (1.9898, 9.0539) ccw
  arc A205 (1.9684, 8.9563) -> (1.6089, 9.0278) centre (0, 0) ccw
  arc A206 (1.5453, 9.0678) -> (1.6089, 9.0278) centre (1.6264, 9.1262) ccw
  arc A207 (1.3034, 9.6968) -> (1.5453, 9.0678) centre (2.6205, 9.8421) ccw
  arc A208 (1.3034, 9.6968) -> (1.1363, 9.8648) centre (1.1146, 9.676) ccw
  arc A209 (1.1363, 9.8648) -> (0.9733, 9.8822) centre (0, 0) ccw
  arc A210 (0.9733, 9.8822) -> (0.81, 9.8969) centre (0, 0) ccw
  arc A211 (0.81, 9.8969) -> (0.6134, 9.7648) centre (0.7945, 9.7075) ccw
  arc A212 (0.2534, 9.195) -> (0.6134, 9.7648) centre (-0.65, 10.1642) ccw
  arc A213 (0.1833, 9.1682) -> (0.2534, 9.195) centre (0.1853, 9.2681) ccw
  arc A214 (0.1833, 9.1682) -> (-0.1833, 9.1682) centre (0, 0) ccw
  arc A215 (-0.2534, 9.195) -> (-0.1833, 9.1682) centre (-0.1853, 9.2681) ccw
  arc A216 (-0.6134, 9.7648) -> (-0.2534, 9.195) centre (0.65, 10.1642) ccw
  arc A217 (-0.6134, 9.7648) -> (-0.81, 9.8969) centre (-0.7945, 9.7075) ccw
  arc A218 (-0.81, 9.8969) -> (-0.9733, 9.8822) centre (0, 0) ccw
  arc A219 (-0.9733, 9.8822) -> (-1.1363, 9.8648) centre (0, 0) ccw
  arc A220 (-1.1363, 9.8648) -> (-1.3034, 9.6968) centre (-1.1146, 9.676) ccw
  arc A221 (-1.5453, 9.0678) -> (-1.3034, 9.6968) centre (-2.6205, 9.8421) ccw
  arc A222 (-1.6089, 9.0278) -> (-1.5453, 9.0678) centre (-1.6264, 9.1262) ccw
  arc A223 (-1.6089, 9.0278) -> (-1.9684, 8.9563) centre (0, 0) ccw
  arc A224 (-2.0424, 8.9689) -> (-1.9684, 8.9563) centre (-1.9898, 9.0539) ccw
  arc A225 (-2.5066, 9.4575) -> (-2.0424, 8.9689) centre (-1.3454, 10.0957) ccw
  arc A226 (-2.5066, 9.4575) -> (-2.7253, 9.5487) centre (-2.6731, 9.366) ccw
  arc A227 (-2.7253, 9.5487) -> (-2.8825, 9.5024) centre (0, 0) ccw
  arc A228 (-2.8825, 9.5024) -> (-3.039, 9.4535) centre (0, 0) ccw
  arc A229 (-3.039, 9.4535) -> (-3.1702, 9.2562) centre (-2.9809, 9.2726) ccw
  arc A230 (-3.2846, 8.5921) -> (-3.1702, 9.2562) centre (-4.4902, 9.1418) ccw
  arc A231 (-3.3392, 8.5404) -> (-3.2846, 8.5921) centre (-3.3756, 8.6335) ccw
  arc A232 (-3.3392, 8.5404) -> (-3.6778, 8.4002) centre (0, 0) ccw
  arc A233 (-3.7529, 8.3981) -> (-3.6778, 8.4002) centre (-3.7179, 8.4918) ccw
  arc A234 (-4.3035, 8.7868) -> (-3.7529, 8.3981) centre (-3.2892, 9.6393) ccw
  arc A235 (-4.3035, 8.7868) -> (-4.5357, 8.8336) centre (-4.449, 8.6645) ccw
  arc A236 (-4.5357, 8.8336) -> (-4.681, 8.7575) centre (0, 0) ccw
  arc A237 (-4.681, 8.7575) -> (-4.8249, 8.679) centre (0, 0) ccw
  arc A238 (-4.8249, 8.679) -> (-4.915, 8.4599) centre (-4.7326, 8.5129) ccw
  arc A239 (-4.8977, 7.7862) -> (-4.915, 8.4599) centre (-6.1874, 8.0901) ccw
  arc A240 (-4.9412, 7.7249) -> (-4.8977, 7.7862) centre (-4.9951, 7.8091) ccw
  arc A241 (-4.9412, 7.7249) -> (-5.2459, 7.5212) centre (0, 0) ccw
  arc A242 (-5.3192, 7.5046) -> (-5.2459, 7.5212) centre (-5.3031, 7.6033) ccw
  arc A243 (-5.935, 7.7784) -> (-5.3192, 7.5046) centre (-5.1065, 8.8124) ccw
  arc A244 (-5.935, 7.7784) -> (-6.1719, 7.779) centre (-6.0538, 7.6301) ccw
  arc A245 (-6.1719, 7.779) -> (-6.2995, 7.676) centre (0, 0) ccw
  arc A246 (-6.2995, 7.676) -> (-6.4254, 7.5709) centre (0, 0) ccw
  arc A247 (-6.4254, 7.5709) -> (-6.4711, 7.3385) centre (-6.3025, 7.4261) ccw
  arc A248 (-6.3226, 6.6811) -> (-6.4711, 7.3385) centre (-7.6468, 6.7276) ccw
  arc A249 (-6.3533, 6.6125) -> (-6.3226, 6.6811) centre (-6.4226, 6.6846) ccw
  arc A250 (-6.3533, 6.6125) -> (-6.6125, 6.3533) centre (0, 0) ccw
  arc A251 (-6.6811, 6.3226) -> (-6.6125, 6.3533) centre (-6.6846, 6.4226) ccw
  arc A252 (-7.3385, 6.4711) -> (-6.6811, 6.3226) centre (-6.7276, 7.6468) ccw
  arc A253 (-7.3385, 6.4711) -> (-7.5709, 6.4254) centre (-7.4261, 6.3025) ccw
  arc A254 (-7.5709, 6.4254) -> (-7.676, 6.2995) centre (0, 0) ccw
  arc A255 (-7.676, 6.2995) -> (-7.779, 6.1719) centre (0, 0) ccw
  arc A256 (-7.779, 6.1719) -> (-7.7784, 5.935) centre (-7.6301, 6.0538) ccw
  arc A257 (-7.5046, 5.3192) -> (-7.7784, 5.935) centre (-8.8124, 5.1065) ccw
  arc A258 (-7.5212, 5.2459) -> (-7.5046, 5.3192) centre (-7.6033, 5.3031) ccw
  arc A259 (-7.5212, 5.2459) -> (-7.7249, 4.9412) centre (0, 0) ccw
  arc A260 (-7.7862, 4.8977) -> (-7.7249, 4.9412) centre (-7.8091, 4.9951) ccw
  arc A261 (-8.4599, 4.915) -> (-7.7862, 4.8977) centre (-8.0901, 6.1874) ccw
  arc A262 (-8.4599, 4.915) -> (-8.679, 4.8249) centre (-8.5129, 4.7326) ccw
  arc A263 (-8.679, 4.8249) -> (-8.7575, 4.681) centre (0, 0) ccw
  arc A264 (-8.7575, 4.681) -> (-8.8336, 4.5357) centre (0, 0) ccw
  arc A265 (-8.8336, 4.5357) -> (-8.7868, 4.3035) centre (-8.6645, 4.449) ccw
  arc A266 (-8.3981, 3.7529) -> (-8.7868, 4.3035) centre (-9.6393, 3.2892) ccw
  arc A267 (-8.4002, 3.6778) -> (-8.3981, 3.7529) centre (-8.4918, 3.7179) ccw
  arc A268 (-8.4002, 3.6778) -> (-8.5404, 3.3392) centre (0, 0) ccw
  arc A269 (-8.5921, 3.2846) -> (-8.5404, 3.3392) centre (-8.6335, 3.3756) ccw
  arc A270 (-9.2562, 3.1702) -> (-8.5921, 3.2846) centre (-9.1418, 4.4902) ccw
  arc A271 (-9.2562, 3.1702) -> (-9.4535, 3.039) centre (-9.2726, 2.9809) ccw
  arc A272 (-9.4535, 3.039) -> (-9.5024, 2.8825) centre (0, 0) ccw
  arc A273 (-9.5024, 2.8825) -> (-9.5487, 2.7253) centre (0, 0) ccw
  arc A274 (-9.5487, 2.7253) -> (-9.4575, 2.5066) centre (-9.366, 2.6731) ccw
  arc A275 (-8.9689, 2.0424) -> (-9.4575, 2.5066) centre (-10.0957, 1.3454) ccw
  arc A276 (-8.9563, 1.9684) -> (-8.9689, 2.0424) centre (-9.0539, 1.9898) ccw
  arc A277 (-8.9563, 1.9684) -> (-9.0278, 1.6089) centre (0, 0) ccw
  arc A278 (-9.0678, 1.5453) -> (-9.0278, 1.6089) centre (-9.1262, 1.6264) ccw
  arc A279 (-9.6968, 1.3034) -> (-9.0678, 1.5453) centre (-9.8421, 2.6205) ccw
  arc A280 (-9.6968, 1.3034) -> (-9.8648, 1.1363) centre (-9.676, 1.1146) ccw
  arc A281 (-9.8648, 1.1363) -> (-9.8822, 0.9733) centre (0, 0) ccw
  arc A282 (-9.8822, 0.9733) -> (-9.8969, 0.81) centre (0, 0) ccw
  arc A283 (-9.8969, 0.81) -> (-9.7648, 0.6134) centre (-9.7075, 0.7945) ccw
  arc A284 (-9.195, 0.2534) -> (-9.7648, 0.6134) centre (-10.1642, -0.65) ccw
  arc A285 (-9.1682, 0.1833) -> (-9.195, 0.2534) centre (-9.2681, 0.1853) ccw
  arc A286 (-9.1682, 0.1833) -> (-9.1682, -0.1833) centre (0, 0) ccw
  arc A287 (-9.195, -0.2534) -> (-9.1682, -0.1833) centre (-9.2681, -0.1853) ccw
  arc A288 (-9.7648, -0.6134) -> (-9.195, -0.2534) centre (-10.1642, 0.65) ccw
  constraints: 576 point on circle, 289 centre point
extrude "Extrusion1" cut sketch "_____6" along normal blind 11
sketch "_____18" plane through (7.5, 0, 0) normal (1, 0, 0) x (0, 0, -1)
  line L0 (0, 0) -> (0, 9.93)
  line L1 (0, 9.93) -> (1.2295, 9.93)
  line L2 (1.2295, 9.93) -> (1.2295, 0)
  line L3 (1.2295, 0) -> (0, 0)
  line L4 (0, 0) -> (0, 9.93)
  constraints: 10 end point
revolve "Revolution2" cut sketch "_____18" angle 360 about axis through (7.5, 0, 0) along (0, -1, 0)
thread "Thread1" size "M3x0.5" class "6H" standard "ISO Metric profile" length 7.93
sketch "_____19" plane through (7.5, 0, 0) normal (1, 0, 0) x (0, 0, -1)
  line L0 (0, 0) -> (8.2565, -5.5168)
  line L1 (8.2565, -5.5168) -> (7.5734, -6.5391)
  line L2 (7.5734, -6.5391) -> (-0.6831, -1.0223)
  line L3 (-0.6831, -1.0223) -> (0, 0)
  line L4 (0, 0) -> (8.2565, -5.5168)
  constraints: 10 end point
revolve "Revolution3" cut sketch "_____19" angle 360 about axis through (7.5, 0, 0) along (0, 0.5555702, 0.8314696)
thread "Thread2" size "M3x0.5" class "6H" standard "ISO Metric profile" length 7.93
ref_plane "C1_XY" through (7.5, 0, 0) normal (1, 0, 0) x (0, 0, -1)
ref_plane "C1_YZ" through (7.5, 0, 0) normal (0, 0, -1) x (0, 1, 0)
ref_plane "C1_ZX" through (7.5, 0, 0) normal (0, 1, 0) x (1, 0, 0)
ref_plane "to_belt_XY" through (7.5, 0, 0) normal (-1, 0, 0) x (0, 0, -1)
ref_plane "to_belt_YZ" through (7.5, 0, 0) normal (0, 0, -1) x (0, -1, 0)
ref_plane "to_belt_ZX" through (7.5, 0, 0) normal (0, -1, 0) x (-1, 0, 0)
ref_plane "to_s1_XY" through (7.5, 2, 0) normal (0, 1, 0) x (1, 0, 0)
ref_plane "to_s1_YZ" through (7.5, 2, 0) normal (1, 0, 0) x (0, 0, -1)
ref_plane "to_s1_ZX" through (7.5, 2, 0) normal (0, 0, -1) x (0, 1, 0)
ref_plane "to_s2_XY" through (7.5, -1.1111, -1.6629) normal (0, -0.5555702, -0.8314696) x (1, 0, 0)
ref_plane "to_s2_YZ" through (7.5, -1.1111, -1.6629) normal (1, 0, 0) x (0, -0.8314696, 0.5555702)
ref_plane "to_s2_ZX" through (7.5, -1.1111, -1.6629) normal (0, -0.8314696, 0.5555702) x (0, -0.5555702, -0.8314696)
body "Solid1"
